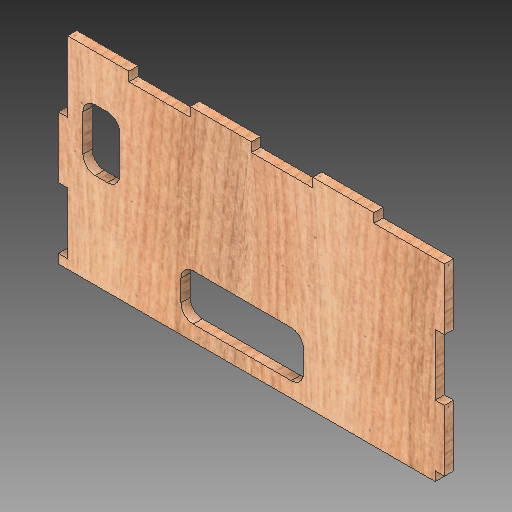
# Autodesk Inventor part: ControlBoxFanFace
Saved by Autodesk Inventor 2018.2 (Build 222227000, 227)
## iProperties
Created: 2018-03-30
Part Number: ControlBoxFanFace
Material: Wood (Birch)
Document SubType Name: Modeling
Designer: Muchen He
Density: 0.55 g/cm^3
Appearance: Birch - Natural Polished
Mass: 11.7422 g
Surface Area: 159.377 cm^2
Volume: 21.3494 cm^3
Author: Muchen He
Autodesk Inventor part; units mm, degrees
ref_plane "YZ Plane" through (0, 0, 0) normal (1, 0, 0) x (0, 1, 0)
ref_plane "XZ Plane" through (0, 0, 0) normal (0, 1, 0) x (-1, 0, 0)
ref_plane "XY Plane" through (0, 0, 0) normal (0, 0, 1) x (1, 0, 0)
sketch "Sketch1" plane through (0, 0, 0) normal (0, 0, 1) x (1, 0, 0)
  line L0 (0, 0) -> (3, 0)
  line L1 (3, 0) -> (123, 0)
  line L2 (0, 0) -> (0, 3)
  line L3 (0, 3) -> (3, 3)
  line L4 (3, 3) -> (3, 23)
  line L5 (3, 23) -> (0, 23)
  line L6 (0, 23) -> (0, 43)
  line L7 (0, 43) -> (3, 43)
  line L8 (3, 43) -> (3, 63)
  line L9 (3, 63) -> (3, 66)
  line L10 (3, 66) -> (23, 66)
  line L11 (23, 66) -> (23, 63)
  line L12 (23, 63) -> (43, 63)
  line L13 (43, 63) -> (43, 66)
  line L14 (43, 66) -> (63, 66)
  line L15 (63, 66) -> (63, 63)
  line L16 (63, 63) -> (83, 63)
  line L17 (83, 63) -> (83, 66)
  line L18 (83, 66) -> (103, 66)
  line L19 (103, 66) -> (103, 63)
  line L20 (103, 63) -> (123, 63)
  line L21 (123, 63) -> (126, 63)
  line L22 (126, 63) -> (126, 43)
  line L23 (126, 43) -> (123, 43)
  line L24 (123, 43) -> (123, 23)
  line L25 (123, 23) -> (126, 23)
  line L26 (126, 23) -> (126, 3)
  line L27 (126, 3) -> (123, 3)
  line L28 (123, 0) -> (123, 3)
  dimension "d0" = 3
  dimension "d1" = 120
  dimension "d2" = 3
  dimension "d3" = 20
  dimension "d4" = 20
  dimension "d5" = 20
  dimension "d6" = 3
  dimension "d7" = 20
  dimension "d8" = 20
  dimension "d9" = 20
  dimension "d10" = 20
  dimension "d11" = 20
  dimension "d12" = 20
  dimension "d13" = 3
  dimension "d14" = 20
  dimension "d15" = 20
  dimension "d16" = 20
  constraints: 58 end point, 23 point on line, 12 perpendicular, 3 vertical alignment, 1 horizontal, 1 horizontal alignment, 1 vertical
  measures "d0" distance of L0.start L0.end
  measures "d1" distance of L0.end L1.end
  measures "d2" distance of L0.start L2.end
  measures "d3" distance of L3.end L4.end
  measures "d4" distance of L5.end L6.end
  measures "d5" distance of L7.end L8.end
  measures "d6" distance of L8.end L9.end
  measures "d7" distance of L9.end L10.end
  measures "d8" distance of L11.end L12.end
  measures "d9" distance of L13.end L14.end
  measures "d10" distance of L15.end L16.end
  measures "d11" distance of L17.end L18.end
  measures "d12" distance of L19.end L20.end
  measures "d13" distance of L20.end L21.end
  measures "d14" distance of L21.end L22.end
  measures "d15" distance of L23.end L24.end
  measures "d16" distance of L25.end L26.end
extrude "Extrusion1" add sketch "Sketch1" along normal blind 3
sketch "Sketch2" plane through (0, 0, 3) normal (0, 0, 1) x (1, 0, 0)
  line L0 (40, 20) -> (80, 20)
  line L1 (80, 20) -> (80, 5)
  line L2 (80, 5) -> (40, 5)
  line L3 (40, 5) -> (40, 20)
  line L4 (0, 0) -> (123, 0) projected
  line L5 (8, 51) -> (20, 51)
  line L6 (20, 51) -> (20, 31)
  line L7 (20, 31) -> (8, 31)
  line L8 (8, 31) -> (8, 51)
  line L9 (43, 63) -> (23, 63) projected
  line L10 (3, 23) -> (3, 3) projected
  dimension "d19" = 40
  dimension "d20" = 15
  dimension "d21" = 5
  dimension "d22" = 40
  dimension "d26" = 12
  dimension "d27" = 20
  dimension "d28" = 12
  dimension "d29" = 5
  constraints: 16 end point, 4 parallel, 2 horizontal, 2 perpendicular
  measures "d19" distance of L1.end L2.end
  measures "d20" distance of L0.end L1.end
  measures "d21" distance between parallel lines of L4 L2
  measures "d22" distance from line of L4.start L3
  measures "d26" distance of L6.end L7.end
  measures "d27" distance of L5.end L6.end
  measures "d28" distance between parallel lines of L9 L5
  measures "d29" distance between parallel lines of L10 L8
extrude "Extrusion2" cut sketch "Sketch2" against normal up to next
fillet "Fillet1" radius 4 8 edges at (20, 31, 1.5) (20, 51, 1.5) (8, 51, 1.5) (8, 31, 1.5) (80, 5, 1.5) (80, 20, 1.5) (40, 20, 1.5) (40, 5, 1.5)
body "Solid1"
